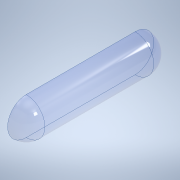
# Autodesk Inventor part: water_hull
Saved by Autodesk Inventor 2020.2 (Build 242310000, 310)
## iProperties
Created: 2020-03-22
Part Number: water_hull
Material: Water
Document SubType Name: Modeling
Designer: agmle
Density: 0.9983 g/cm^3
Appearance: Tropical Blue
Author: agmle
Autodesk Inventor part; units mm, degrees
ref_plane "YZ Plane" through (0, 0, 0) normal (1, 0, 0) x (0, 1, 0)
ref_plane "XZ Plane" through (0, 0, 0) normal (0, 1, 0) x (-1, 0, 0)
ref_plane "XY Plane" through (0, 0, 0) normal (0, 0, 1) x (1, 0, 0)
sketch "Sketch1" plane through (0, 0, 0) normal (1, 0, 0) x (0, 1, 0)
  line L0 (0, 429.3616) -> (0, -429.3616)
  arc A0 (0, 429.3616) -> (-109.5375, 319.8241) centre (0, 319.8241) ccw
  arc A1 (-109.5375, -319.8241) -> (0, -429.3616) centre (0, -319.8241) ccw
  line L1 (-109.5375, -319.8241) -> (-109.5375, 319.8241)
  point P0 (0, 0)
  point P1 (0, 0)
  dimension "d0" = 109.5375
  dimension "d1" = 639.6482
  constraints: 4 end point, 4 point on circle, 2 centre point, 2 point on line, 2 tangent, 1 coincident, 1 midpoint, 1 parallel, 1 vertical
  measures "d0" distance between parallel lines of L1 L0
  measures "d1" distance of L1.start L1.end
revolve "Revolution1" add sketch "Sketch1" angle 180 about axis through (0, 0, 429.3616) along (0, 0, 1)
equation "\"d0\" = 0.5 * hull_od"
equation "\"hull_od\" = 219.075"
equation "\"hull_id\" = 201.7268"
equation "\"hull_wall\" = 8.6741"
equation "\"hull_length\" = 609.6"
equation "\"hull_spacing\" = 390.525"
equation "\"impeller_od\" = 76.2"
equation "\"impeller_clearance\" = 0.5"
equation "\"impeller_shaft_id\" = 3.175"
equation "\"impeller_shaft_od\" = 5.715"
equation "\"impeller_shaft_support\" = 3.175"
equation "\"impeller_intake_od\" = 19.05"
equation "\"impeller_vane_thick\" = 2"
equation "\"impeller_vane_inner_rad\" = 3.175"
equation "\"impeller_vane_outer_rad\" = 0.37206"
equation "\"magnet_od\" = 5.95"
equation "\"magnet_clearance\" = 0.25"
equation "\"magnet_rad\" = 0.25"
equation "\"magnet_circle_offset\" = 3.175"
equation "\"motor_shaft_od\" = 12.7"
equation "\"motor_shaft_length\" = 31.75"
equation "\"motor_shaft_key\" = 3.048"
body "Solid1"
